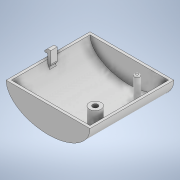
# Autodesk Inventor part: base_snap_test
Saved by Autodesk Inventor 2021 (Build 250183000, 183)
## iProperties
Created: 2023-08-20
Part Number: base_snap_test
Material: Genérico
Document SubType Name: Modeling
Designer: Sergio
Density: 1 g/cm^3
Appearance: Valor por defecto
Author: Sergio
Autodesk Inventor part; units mm, degrees
ref_plane "YZ Plane" through (0, 0, 0) normal (1, 0, 0) x (0, 1, 0)
ref_plane "XZ Plane" through (0, 0, 0) normal (0, 1, 0) x (-1, 0, 0)
sketch "Boceto1" plane through (0, 0, 0) normal (0, 0, 1) x (1, 0, 0)
  line L0 (0, 4) -> (-2, 4)
  line L1 (2.5, 4) -> (2.5, 7)
  line L2 (2.5, 7) -> (0, 7)
  line L3 (0, 7) -> (-2, 5)
  line L4 (0, -5.5) -> (0, 0)
  line L5 (2.5, 4) -> (2.5, 0)
  line L6 (2.5, 0) -> (2.5, -2.1716)
  line L7 (1.9142, -3.5858) -> (1.1716, -4.3284)
  line L8 (0, 4) -> (0.25, 4)
  line L9 (0.25, 4) -> (0.25, 0)
  line L10 (-2, 4) -> (-2, 5)
  arc A0 (1.9142, -3.5858) -> (2.5, -2.1716) centre (0.5, -2.1716) ccw
  line L11 (0, 0) -> (0, -10.5)
  arc A1 (1.1716, -4.3284) -> (0, -7.1569) centre (4, -7.1569) ccw
  line L12 (0, 0) -> (2.5, 0)
  point P0 (2.5, -3)
  dimension "d0" = 2.5
  dimension "d2" = 3
  dimension "d3" = 4
  dimension "d4" = 4
  dimension "d27" = 0.25
  dimension "d28" = 45
  dimension "d29" = 2
  dimension "d30" = 1
  dimension "d31" = 3
  dimension "d32" = 45
  dimension "d33" = 2
  dimension "d34" = 5
  dimension "d35" = 4
  constraints: 26 end point, 7 point on line, 4 point on circle, 4 tangent, 4 vertical, 2 centre point, 2 perpendicular, 1 horizontal
  measures "d0" distance of L4.end L5.end
  measures "d2" distance of L1.start L1.end
  measures "d3" distance of L4.end L0.start
  measures "d4" distance of L5.end L1.start
  measures "d27" distance of L0.start L8.end
  measures "d28" angle of L0 L3
  measures "d29" distance of L0.start L0.end
  measures "d30" distance of L0.end L3.end
  measures "d31" distance of L5.end point (2.5, -3)
  measures "d32" angle of L4 L7
  measures "d33" radius of A0
  measures "d34" distance of L4.start L11.end
  measures "d35" radius of A1
sketch "Boceto2" plane through (0, 0, 0) normal (0, 1, 0) x (-1, 0, 0)
  line L0 (0, 0) -> (2, 0)
  line L1 (0, 0) -> (-30, 0)
  line L2 (-62, -32) -> (2, -32)
  line L3 (2, -32) -> (2, 32)
  line L4 (2, 32) -> (-62, 32)
  line L5 (-62, 32) -> (-62, -32)
  line L6 (-62, -32) -> (2, 32) construction
  line L7 (2, -32) -> (-62, 32) construction
  dimension "d6" = 2
  dimension "d7" = 30
  dimension "d8" = 64
  dimension "d9" = 64
  constraints: 16 end point, 3 horizontal, 2 midpoint, 2 parallel, 1 perpendicular
  measures "d6" distance of L0.start L0.end
  measures "d7" distance of L0.start L1.end
  measures "d8" distance of L4.end L3.end
  measures "d9" distance of L3.end L2.end
extrude "Extrusión1" add sketch "Boceto2" along normal blind 20 and the other way blind 20
shell "Vaciado1" thickness 2 removed faces 0
ref_plane "Plano de trabajo2" through (0, 0, 0) normal (0, -1, 0) x (1, 0, 0)
sketch "Boceto3" plane through (0, 0, 0) normal (0, -1, 0) x (1, 0, 0)
  line L0 (60, 30) -> (60, -30) projected
  line L1 (60, 0) -> (50, 0)
  line L2 (50, 0) -> (50, -16)
  line L3 (50, 0) -> (50, 16)
  circle A0 centre (50, -16) radius 2
  circle A1 centre (50, 16) radius 4.5
  point P0 (0, 0)
  dimension "d20" = 10
  dimension "d21" = 16
  dimension "d22" = 16
  dimension "d23" = 4
  dimension "d24" = 9
  constraints: 6 end point, 2 centre point, 2 coincident, 2 vertical, 1 horizontal, 1 midpoint
  measures "d20" distance of L1.start L1.end
  measures "d21" distance of L1.end L2.end
  measures "d22" distance of L1.end L3.end
  measures "d23" diameter of A0
  measures "d24" diameter of A1
extrude "Extrusión2" add sketch "Boceto3" along normal through all
sketch "Boceto4" plane through (0, 0, 0) normal (0, -1, 0) x (1, 0, 0)
  line L0 (81.7327, 42.0826) -> (-20.271, 42.0826)
  line L1 (-20.271, 42.0826) -> (-20.271, -44.6773)
  line L2 (-20.271, -44.6773) -> (81.7327, -44.6773)
  line L3 (81.7327, -44.6773) -> (81.7327, 42.0826)
  point P0 (0, 0)
  constraints: 8 end point, 2 parallel, 1 horizontal, 1 perpendicular
extrude "Extrusión3" cut sketch "Boceto4" against normal through all
extrude "Extrusión4" add sketch "Boceto1" against normal mid plane 5
sketch "Boceto5" plane through (50, 0, -16) normal (0, 1, 0) x (1, 0, 0)
  circle A0 centre (0, 0) radius 2 projected
  circle A1 centre (0, 0) radius 2
  point P0 (-50, -16)
  dimension "d40" = 4
  constraints: 1 centre point, 1 coincident
  measures "d40" diameter of A1
extrude "Extrusión5" add sketch "Boceto5" along normal blind 6
fillet "Empalme1" radius 1 1 edges at (48, 6, -16)
sketch "Boceto6" plane through (50, 0, 16) normal (0, 1, 0) x (1, 0, 0)
  circle A0 centre (0, 0) radius 4.5
  point P0 (-50, 16)
  dimension "d44" = 9
  constraints: 1 centre point
  measures "d44" diameter of A0
extrude "Extrusión6" add sketch "Boceto6" along normal blind 1
sketch "Boceto7" plane through (50, 1, 16) normal (0, 1, 0) x (1, 0, 0)
  circle A0 centre (0, 0) radius 2
  point P0 (-50, 16)
  dimension "d47" = 4
  constraints: 1 centre point
  measures "d47" diameter of A0
hole "Agujero1" at (50, 1, 16) direction (0, -1, 0) diameter 4 depth 10
thread "Rosca1" size "M4x0.7" class "6H" standard "ANSI Metric M Profile" full length
sketch "Boceto8" plane through (0, 0, 0) normal (0, 0, 1) x (1, 0, 0)
  line L0 (0, 0) -> (60, 0) projected
  line L1 (-2, 0) -> (-2, -20) projected
  line L2 (0, 0) -> (-2, 0)
  line L3 (62, 0) -> (-2, 0) projected
  line L4 (-2, 0) -> (62, 0)
  ellipse E0 centre (30, 0) end of major axis (-2, 0) minor radius 20 (-2, 0) -> (62, 0) ccw
  line L5 (-17, 0) -> (77, 0)
  spline S0 degree 5 poles (-17, 0) (-17.0001, -3.7485) (-16.3619, -7.497) (-15.0818, -11.0973) (-11.4861, -17.6731) (-6.2212, -23.0069) (-3.3113, -25.2996) (2.948, -29.2454) (9.8361, -31.95) (13.3871, -33.0146) (20.6763, -34.6099) (28.1196, -35.1321) (31.8804, -35.1321) (39.3237, -34.6099) (46.6129, -33.0146) (50.1639, -31.95) (57.052, -29.2454) (63.3113, -25.2996) (66.2212, -23.0069) (71.4861, -17.6731) (75.0818, -11.0973) (76.3619, -7.497) (77.0001, -3.7485) (77, 0) knots 0 0 0 0 0 0 0.144277 0.144277 0.144277 0.285695 0.285695 0.285695 0.427847 0.427847 0.427847 0.572153 0.572153 0.572153 0.714305 0.714305 0.714305 0.855723 0.855723 0.855723 1 1 1 1 1 1
  point P0 (-2, 10)
  point P1 (62, 10)
  dimension "d59" = 20
  dimension "d60" = 15
  constraints: 6 end point, 3 horizontal, 2 point on line, 1 collinear, 1 midpoint, 9 other
extrude "Extrusión7" cut sketch "Boceto8" along normal through all both and the other way through all contours E0 L5 S0
sketch "Boceto9" plane through (0, 0, 0) normal (0, 0, 1) x (1, 0, 0)
  line L0 (0, 0) -> (60, 0)
  line L1 (-2, 0) -> (-2, -20)
  line L2 (0, 0) -> (-2, 0)
  line L3 (62, 0) -> (-2, 0)
  line L4 (-2, 0) -> (62, 0)
  ellipse E0 centre (30, 0) end of major axis (-2, 0) minor radius 20 (-2, 0) -> (62, 0) ccw
  ellipse E1 centre (30, 0) end of major axis (0, 0) minor radius 18 (0, 0) -> (60, 0) ccw
  point P0 (0, 0)
  point P1 (-2, 10)
  point P2 (62, 10)
  dimension "d63" = 20
  constraints: 10 end point, 2 horizontal, 1 collinear, 1 midpoint, 8 other
extrude "Extrusión8" add sketch "Boceto9" along normal through all both and the other way through all contours E1 L3 E0 L2
fillet "Empalme2" radius 2 2 edges at (0.9715, -4.5437, 1.25) (0.9715, -4.5437, -1.25)
equation "\"d0\" = sf_head_width - sf_head_grip_width"
equation "\"d2\" = sf_head_height"
equation "\"d3\" = d4"
equation "\"d4\" = sf_lenght - sf_head_height"
equation "\"d27\" = sf_head_offset"
equation "\"d28\" = sf_head_angle"
equation "\"d29\" = sf_head_grip_width"
equation "\"d31\" = sf_base"
equation "\"d8\" = 2 * d6 + 2 * d7"
equation "\"d9\" = 2 * d6 + 2 * d7"
equation "\"d21\" = 0.25 * d9"
equation "\"d22\" = 0.25 * d9"
equation "\"d23\" = gj_d"
equation "\"d24\" = screwJ_base_D"
equation "\"d38\" = sf_thikness"
equation "\"d40\" = gj_d"
equation "\"d41\" = gj_out_section"
equation "\"d44\" = screwJ_base_D"
equation "\"d45\" = 0.5 * thikness"
equation "\"cell_z_space\" = 5"
equation "\"d47\" = screw_d"
equation "\"d53\" = screw_lenght - thikness"
equation "\"sf_lenght\" = 7"
equation "\"sf_base\" = 3"
equation "\"sf_head_height\" = 3"
equation "\"sf_head_offset\" = 0.25"
equation "\"sf_head_angle\" = 45deg"
equation "\"sf_head_width\" = 4.5"
equation "\"sf_head_grip_width\" = 2"
equation "\"thikness\" = 2"
equation "\"offset\" = 1"
equation "\"r1\" = 3.5"
equation "\"r2o\" = 60.25"
equation "\"delta_y\" = 6"
equation "\"wire_d\" = 1"
equation "\"width_ang_spring\" = 5"
equation "\"spring_int_diam\" = 8.5"
equation "\"spring_ext_diam\" = 10.5"
equation "\"r3\" = 8.25"
equation "\"r3R\" = 4.75"
equation "\"r3T\" = 6.74537"
equation "\"alpha\" = 54.847297deg"
equation "\"alpha2\" = 270deg"
equation "\"theta3_recogido\" = 305.152703deg"
equation "\"delta_theta_3\" = 45deg"
equation "\"joint_width\" = 12"
equation "\"joint_radius\" = 7.75"
equation "\"shaft_width\" = 15"
equation "\"shaft_joint_diameter\" = 3.875"
equation "\"separation_space\" = 0.5"
equation "\"height_finger\" = 42"
equation "\"cell_screw_head_diameter\" = 4"
equation "\"cell_screw_diameter\" = 2"
equation "\"cell_space\" = 2"
equation "\"cell_width\" = 6"
equation "\"cell_theta_position\" = 60deg"
equation "\"cell_thikness\" = 1"
equation "\"cell_lenght\" = 37"
equation "\"wire_D\" = 3.5"
equation "\"width_link\" = 8"
equation "\"Dt\" = 1.05972"
equation "\"Djoint_shaft\" = 4"
equation "\"shaft_x\" = -0.44028"
equation "\"shaft_y\" = 6.5"
equation "\"lenght_body_link\" = 185.5"
equation "\"lenght_bar_support\" = 202"
equation "\"trigger_offset\" = 2"
equation "\"m2_theta2o\" = 107deg"
equation "\"m2_r2\" = 28"
equation "\"e\" = 9"
equation "\"So\" = 17"
equation "\"m2_theta3o\" = -30deg"
equation "\"m2_r3\" = 19.75"
equation "\"m2_delta_theta1\" = 15deg"
equation "\"m2_theta3f\" = -60deg"
equation "\"trigger_thumb_lenght\" = 6"
equation "\"width_r12\" = 8"
equation "\"m2_r1\" = 25.2"
equation "\"r3_thikness\" = 3.5"
equation "\"t_thikness\" = 3"
equation "\"tg_width\" = 4"
equation "\"pivot_screw_d\" = 4"
equation "\"pivot_diameter\" = 7"
equation "\"sj_diam_shaft\" = 6"
equation "\"sj_groove\" = 2"
equation "\"sj_groove_deep\" = 7"
equation "\"sj_head_D\" = 7"
equation "\"sj_head_d\" = 4.7464"
equation "\"sj_head_height\" = 5"
equation "\"sf_thikness\" = 5"
equation "\"screw_Dhead\" = 8"
equation "\"screw_d\" = 4"
equation "\"screw_lenght\" = 12"
equation "\"screwJ_base_D\" = 9"
equation "\"screwJ_top_D\" = 13"
equation "\"gj_D\" = 8"
equation "\"gj_d\" = 4"
equation "\"gj_out_section\" = 6"
